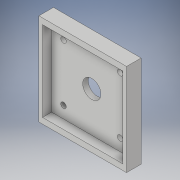
# Autodesk Inventor part: RollMotorMount
Saved by Autodesk Inventor 2019 (Build 230136000, 136)
## iProperties
Created: 2018-05-28
Part Number: RollMotorMount
Material: Generic
Document SubType Name: Modeling
Designer: samps
Density: 1 g/cm^3
Appearance: Default
Author: samps
Autodesk Inventor part; units mm, degrees
ref_plane "YZ Plane" through (0, 0, 0) normal (1, 0, 0) x (0, 1, 0)
ref_plane "XZ Plane" through (0, 0, 0) normal (0, 1, 0) x (-1, 0, 0)
ref_plane "XY Plane" through (0, 0, 0) normal (0, 0, 1) x (1, 0, 0)
sketch "Sketch1" plane through (0, 0, 0) normal (0, 0, 1) x (1, 0, 0)
  line L0 (0, 0) -> (22, 0)
  line L1 (22, 0) -> (22, 22)
  line L2 (22, 22) -> (-22, 22)
  line L3 (-22, 22) -> (-22, -22)
  line L4 (-22, -22) -> (22, -22)
  line L5 (22, -22) -> (22, 22)
  line L6 (-22, 22) -> (-22, 25.175)
  line L7 (-22, 25.175) -> (-25.175, 25.175)
  line L8 (22, -22) -> (25.175, -22)
  line L9 (25.175, -22) -> (25.175, -25.175)
  line L10 (-25.175, 25.175) -> (25.175, 25.175)
  line L11 (25.175, 25.175) -> (25.175, -25.175)
  line L12 (25.175, -25.175) -> (-25.175, -25.175)
  line L13 (-25.175, -25.175) -> (-25.175, 25.175)
  dimension "d0" = 22
  dimension "d1" = 22
  dimension "d2" = 44
  dimension "d3" = 44
  dimension "d4" = 3.175
  dimension "d5" = 3.175
  dimension "d6" = 3.175
  dimension "d7" = 3.175
  constraints: 28 end point, 5 perpendicular, 4 horizontal, 4 parallel, 1 vertical
  measures "d0" distance of L0.start L0.end
  measures "d1" distance of L0.end L1.end
  measures "d2" distance of L4.end L3.end
  measures "d3" distance of L3.end L2.end
  measures "d4" distance of L2.end L6.end
  measures "d5" distance of L6.end L7.end
  measures "d6" distance of L4.end L8.end
  measures "d7" distance of L8.end L9.end
extrude "Extrusion1" add sketch "Sketch1" along normal blind 8 contours L1 L2 L6 L10 L11 L8 L5 | L8 L9 L12 L13 L7 L6 L3 L4
sketch "Sketch2" plane through (0, 0, 0) normal (0, 0, -1) x (-1, 0, 0)
  line L0 (22, 22) -> (-22, 22) projected
  line L1 (-22, 22) -> (-22, -22) projected
  line L2 (22, 22) -> (-22, 22)
  line L3 (-22, 22) -> (-22, -22)
  line L4 (-22, -22) -> (22, -22)
  line L5 (22, -22) -> (22, 22)
  point P0 (0, 0)
  constraints: 8 end point, 2 parallel, 1 horizontal, 1 perpendicular
extrude "Extrusion2" add sketch "Sketch2" against normal blind 3
sketch "Sketch3" plane through (0, 0, 3) normal (0, 0, 1) x (1, 0, 0)
  line L0 (-22, 22) -> (22, 22) projected
  line L1 (-22, 22) -> (0, 22)
  point P0 (0, 0)
  point P1 (0, 0)
  constraints: 2 end point, 1 coincident, 1 midpoint
hole "Hole1" at (0, 0, 3) direction (0, 0, -1) diameter 10 end through all
sketch "Sketch4" plane through (0, 0, 3) normal (0, 0, 1) x (1, 0, 0)
  line L0 (0, 0) -> (0, 15.5)
  line L1 (0, 15.5) -> (15.5, 15.5)
  line L2 (15.5, 15.5) -> (-15.5, 15.5)
  line L3 (-15.5, 15.5) -> (-15.5, -15.5)
  line L4 (-15.5, -15.5) -> (15.5, -15.5)
  line L5 (15.5, -15.5) -> (15.5, 15.5)
  dimension "d19" = 15.5
  dimension "d20" = 15.5
  dimension "d21" = 31
  dimension "d22" = 31
  constraints: 12 end point, 2 parallel, 2 perpendicular, 1 horizontal, 1 vertical
  measures "d19" distance of L0.start L0.end
  measures "d20" distance of L0.end L1.end
  measures "d21" distance of L4.end L3.end
  measures "d22" distance of L3.end L2.end
hole "Hole2" at (-15.5, 15.5, 3) at (15.5, 15.5, 3) at (15.5, -15.5, 3) at (-15.5, -15.5, 3) direction (0, 0, -1) diameter 3 end through all
sketch "Sketch5" plane through (0, 0, 8) normal (0, 0, 1) x (1, 0, 0)
  line L0 (22, 22) -> (22, -22) projected
  line L1 (22, -22) -> (22, -25.175)
  line L2 (-25.175, -25.175) -> (25.175, -25.175) projected
  line L3 (22, -25.175) -> (24, -25.175)
  line L4 (22, -22) -> (-22, -22) projected
  line L5 (-22, -22) -> (-22, -25.175)
  line L6 (-22, -25.175) -> (-24, -25.175)
  line L7 (25.175, -25.175) -> (25.175, 25.175) projected
  line L8 (24, -25.175) -> (25.175, -25.175)
  line L9 (25.175, -25.175) -> (25.175, 25.175)
  line L10 (25.175, 25.175) -> (24, 25.175)
  line L11 (24, 25.175) -> (24, -25.175)
  line L12 (25.175, 25.175) -> (-25.175, 25.175) projected
  line L13 (-24, -25.175) -> (-25.175, -25.175)
  line L14 (-25.175, -25.175) -> (-25.175, 25.175)
  line L15 (-25.175, 25.175) -> (-24, 25.175)
  line L16 (-24, 25.175) -> (-24, -25.175)
  point P0 (0, 0)
  dimension "d30" = 2
  dimension "d31" = 2
  constraints: 24 end point, 4 parallel, 3 horizontal, 3 perpendicular, 3 point on line, 1 vertical
  measures "d30" distance of L1.end L3.end
  measures "d31" distance of L5.end L6.end
extrude "Extrusion3" cut sketch "Sketch5" against normal blind 8 contours L11 L10 L7 L2 | L2 L14 L12 L16
body "Solid1"
